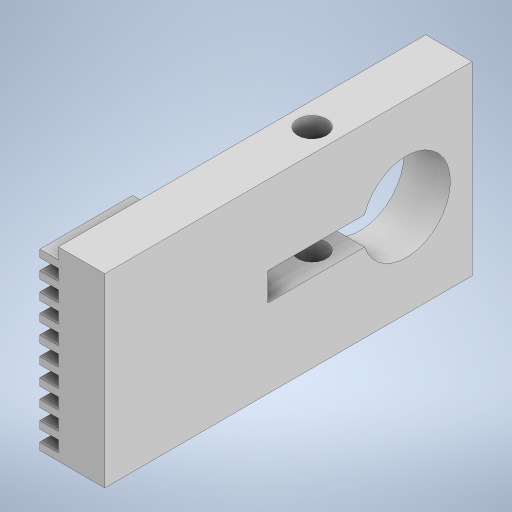
# Autodesk Inventor part: teethset
Saved by Autodesk Inventor 2023 (Build 270158000, 158)
## iProperties
Created: 2025-10-02
Part Number: teethset
Material: Generic
Document SubType Name: Modeling
Designer: ptato_qo49uko
Density: 1 g/cm^3
Appearance: Default
Author: ptato_qo49uko
Autodesk Inventor part; units mm, degrees
ref_plane "YZ Plane" through (0, 0, 0) normal (1, 0, 0) x (0, 1, 0)
ref_plane "XZ Plane" through (0, 0, 0) normal (0, 1, 0) x (-1, 0, 0)
ref_plane "XY Plane" through (0, 0, 0) normal (0, 0, 1) x (1, 0, 0)
sketch "Sketch1" plane through (0, 0, 0) normal (0, 0, 1) x (1, 0, 0)
  line L0 (-2.5, 15.5) -> (2.5, 15.5)
  line L1 (2.5, 15.5) -> (2.5, -4.5)
  line L2 (2.5, -4.5) -> (-2.5, -4.5)
  line L3 (-2.5, -4.5) -> (-2.5, 15.5)
  point P0 (0, 0)
  dimension "d0" = 5
  dimension "d1" = 20
  constraints: 8 end point, 2 parallel, 1 horizontal, 1 perpendicular
  measures "d0" distance of L1.end L2.end
  measures "d1" distance of L0.end L1.end
extrude "Extrusion1" add sketch "Sketch1" along normal blind 40
sketch "Sketch3" plane through (-2.5, -4.5, 0) normal (-1, 0, 0) x (0, 0, 1)
  line L0 (0, 0) -> (0, 20) projected
  line L1 (0, 10) -> (2.5, 10)
  line L2 (2.5, 10) -> (7.5, 10)
  circle A0 centre (7.5, 10) radius 4.75
  point P0 (0, 4.5)
  dimension "d7" = 2.5
  dimension "d38" = 5
  dimension "d39" = 9.5
  constraints: 4 end point, 2 horizontal, 1 centre point, 1 coincident, 1 midpoint
  measures "d7" distance of L1.start L1.end
  measures "d38" distance of L1.end L2.end
  measures "d39" diameter of A0
extrude "Extrusion2" cut sketch "Sketch3" against normal blind 8
sketch "Sketch4" plane through (-2.5, -4.5, 0) normal (-1, 0, 0) x (0, 0, 1)
  line L0 (40, 0) -> (40, 20) projected
  line L1 (40, 0) -> (30, 0)
  line L2 (30, 0) -> (30, 0.8)
  line L3 (30, 0.8) -> (40, 0.8)
  line L4 (40, 0.8) -> (40, 0)
  line L5 (40, 0.8) -> (40, 2)
  line L6 (40, 2) -> (30, 2)
  line L7 (30, 2) -> (30, 2.8)
  line L8 (30, 2.8) -> (40, 2.8)
  line L9 (40, 2.8) -> (40, 2)
  line L10 (40, 2.8) -> (40, 4)
  line L11 (40, 4) -> (30, 4)
  line L12 (30, 4) -> (30, 4.8)
  line L13 (30, 4.8) -> (40, 4.8)
  line L14 (40, 4.8) -> (40, 4)
  line L15 (40, 4.8) -> (40, 6)
  line L16 (40, 6) -> (30, 6)
  line L17 (30, 6) -> (30, 6.8)
  line L18 (30, 6.8) -> (40, 6.8)
  line L19 (40, 6.8) -> (40, 6)
  line L20 (40, 6.8) -> (40, 8)
  line L21 (40, 8) -> (30, 8)
  line L22 (30, 8) -> (30, 8.8)
  line L23 (30, 8.8) -> (40, 8.8)
  line L24 (40, 8.8) -> (40, 8)
  line L25 (40, 8.8) -> (40, 10)
  line L26 (40, 10) -> (30, 10)
  line L27 (30, 10) -> (30, 10.8)
  line L28 (30, 10.8) -> (40, 10.8)
  line L29 (40, 10.8) -> (40, 10)
  line L30 (40, 10.8) -> (40, 12)
  line L31 (40, 12) -> (30, 12)
  line L32 (30, 12) -> (30, 12.8)
  line L33 (30, 12.8) -> (40, 12.8)
  line L34 (40, 12.8) -> (40, 12)
  line L35 (40, 12.8) -> (40, 14)
  line L36 (40, 14) -> (30, 14)
  line L37 (30, 14) -> (30, 14.8)
  line L38 (30, 14.8) -> (40, 14.8)
  line L39 (40, 14.8) -> (40, 14)
  line L40 (40, 14.8) -> (40, 16)
  line L41 (40, 16) -> (30, 16)
  line L42 (30, 16) -> (30, 16.8)
  line L43 (30, 16.8) -> (40, 16.8)
  line L44 (40, 16.8) -> (40, 16)
  line L45 (40, 16.8) -> (40, 18)
  line L46 (40, 18) -> (30, 18)
  line L47 (30, 18) -> (30, 18.8)
  line L48 (30, 18.8) -> (40, 18.8)
  line L49 (40, 18.8) -> (40, 18)
  point P0 (0, 4.5)
  dimension "d12" = 10
  dimension "d13" = 0.8
  dimension "d14" = 1.2
  dimension "d15" = 0.8
  dimension "d16" = 1.2
  dimension "d17" = 0.8
  dimension "d18" = 1.2
  dimension "d19" = 0.8
  dimension "d20" = 1.2
  dimension "d21" = 0.8
  dimension "d22" = 1.2
  dimension "d29" = 0.8
  dimension "d30" = 1.2
  dimension "d31" = 0.8
  dimension "d32" = 1.2
  dimension "d33" = 0.8
  dimension "d34" = 1.2
  dimension "d35" = 0.8
  dimension "d36" = 1.2
  dimension "d37" = 0.8
  constraints: 98 end point, 20 parallel, 10 horizontal, 10 perpendicular, 10 other
  measures "d12" distance of L2.end L3.end
  measures "d13" distance of L1.end L2.end
  measures "d14" distance of L3.end L5.end
  measures "d15" distance of L6.end L7.end
  measures "d16" distance of L8.end L10.end
  measures "d17" distance of L11.end L12.end
  measures "d18" distance of L13.end L15.end
  measures "d19" distance of L16.end L17.end
  measures "d20" distance of L18.end L20.end
  measures "d21" distance of L21.end L22.end
  measures "d22" distance of L23.end L25.end
  measures "d29" distance of L26.end L27.end
  measures "d30" distance of L28.end L30.end
  measures "d31" distance of L31.end L32.end
  measures "d32" distance of L33.end L35.end
  measures "d33" distance of L36.end L37.end
  measures "d34" distance of L38.end L40.end
  measures "d35" distance of L41.end L42.end
  measures "d36" distance of L43.end L45.end
  measures "d37" distance of L46.end L47.end
extrude "Extrusion3" add sketch "Sketch4" along normal blind 2
sketch "Sketch5" plane through (-2.5, -4.5, 0) normal (-1, 0, 0) x (0, 0, 1)
  circle A0 centre (7.5, 10) radius 4.75 projected
  line L0 (12.4308, 11.5) -> (18, 11.5)
  line L1 (22.4308, 8.5) -> (22.4308, 11.5)
  line L2 (22.4308, 11.5) -> (18, 11.5)
  line L3 (22.4308, 8.5) -> (11.2154, 8.5)
  line L4 (11.2154, 8.5) -> (11.2154, 11.5)
  line L5 (11.2154, 11.5) -> (12.4308, 11.5)
  point P0 (0, 4.5)
  constraints: 12 end point, 2 perpendicular, 1 collinear, 1 horizontal, 1 vertical
extrude "Extrusion4" cut sketch "Sketch5" against normal blind 40 contours A0 L3 L4 L5 | A0 L5 L0 L2 L1 L3 picked at (11.5603, 10)
sketch "Sketch6" plane through (-2.5, 15.5, 0) normal (0, 1, 0) x (1, 0, 0)
  line L0 (0, 0) -> (0, -40) projected
  line L1 (0, -15.1532) -> (2.5, -15.1532)
  point P0 (2.5, 0)
  constraints: 2 end point, 1 horizontal, 1 point on line
hole "Hole1" at (0, 15.5, 15.1532) direction (0, -1, 0) diameter 3.1 depth 49.5
sketch "Sketch7" plane through (0, 0, 0) normal (0, 0, -1) x (-1, 0, 0)
  line L0 (-2.5, -4.5) -> (-2.5, 15.5) projected
  line L1 (-2.5, 15.5) -> (2.5392, 15.5)
  line L2 (2.5392, 15.5) -> (2.5392, -4.5)
  line L3 (2.5392, -4.5) -> (-2.5, -4.5)
  line L4 (-2.5, -4.5) -> (-2.5, 15.5)
  point P0 (0, 0)
  constraints: 8 end point, 2 parallel, 1 horizontal, 1 perpendicular
extrude "Extrusion5" cut sketch "Sketch7" against normal blind 0.4
body "Solid1"
